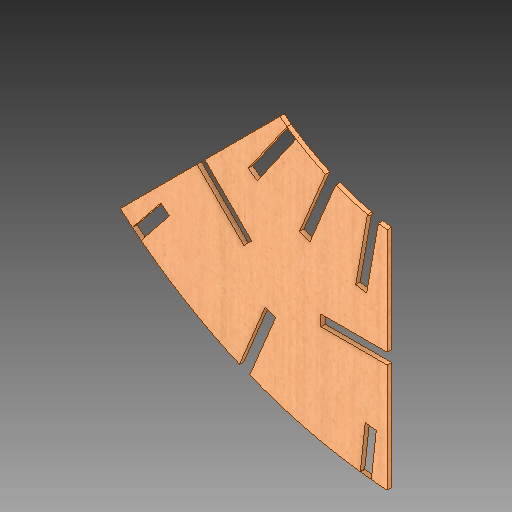
# Autodesk Inventor part: internalSupportTop5
Saved by Autodesk Inventor 2019 (Build 230136000, 136)
## iProperties
Company: FABLAB Torino
Created: 2019-01-11
Part Number: internalSupportTop5
Material: Wood (Cherry)
Document SubType Name: Modeling
Designer: Giancarlo
Density: 0.63 g/cm^3
Appearance: Cherry - Natural Low Gloss
Description: MultiLayer 10mm
Author: Giancarlo
Title: La Panca - Flower Vase
Subject: Construction MOld
Autodesk Inventor part; units mm, degrees
ref_plane "YZ Plane" through (0, 0, 0) normal (1, 0, 0) x (0, 1, 0)
ref_plane "XZ Plane" through (0, 0, 0) normal (0, 1, 0) x (-1, 0, 0)
ref_plane "Work Plane1" through (0, 0, 0) normal (0, 0, 1) x (1, 0, 0)
sketch "Sketch1" plane through (0, 0, 0) normal (0, 0, 1) x (1, 0, 0)
  line L0 (13.372447, 117.409014) -> (-9.931154, 61.149144)
  line L1 (13.372447, 117.409014) -> (4.133652, 121.235848)
  line L2 (-19.16995, 64.975978) -> (4.133652, 121.235848)
  line L3 (-9.931154, 61.149144) -> (-19.16995, 64.975978)
  line L4 (-22.457521, 135.166057) -> (-57.338279, 85.250516)
  line L5 (-22.457521, 135.166057) -> (-30.654475, 140.894052)
  line L6 (-65.535233, 90.978511) -> (-30.654475, 140.894052)
  line L7 (-57.338279, 85.250516) -> (-65.535233, 90.978511)
  line L8 (51.895734, 106.882533) -> (41.300176, 46.916168)
  line L9 (51.895734, 106.882533) -> (42.048271, 108.622498)
  line L10 (31.452714, 48.656133) -> (42.048271, 108.622498)
  line L11 (41.300176, 46.916168) -> (31.452714, 48.656133)
  line L12 (59.884796, 0) -> (0, 0)
  line L13 (59.884796, 0) -> (59.884796, 10)
  line L14 (0, 10) -> (59.884796, 10)
  line L15 (0, 0) -> (0, 10)
  line L16 (32.552055, -95.175797) -> (40.182275, -56.162387)
  line L17 (32.552055, -95.175797) -> (42.366116, -97.095226)
  line L18 (49.996336, -58.081815) -> (42.366116, -97.095226)
  line L19 (40.182275, -56.162387) -> (49.996336, -58.081815)
  line L20 (-81.40859, -85.281526) -> (-58.104996, -29.021673) construction
  line L21 (-81.40859, -85.281526) -> (-72.169794, -89.10836) construction
  line L22 (-48.8662, -32.848507) -> (-72.169794, -89.10836) construction
  line L23 (-58.104996, -29.021673) -> (-48.8662, -32.848507) construction
  line L24 (-167.86588, -9.726604) -> (-145.674595, 23.255452)
  line L25 (-167.86588, -9.726604) -> (-159.56905, -15.308952)
  line L26 (-137.377765, 17.673104) -> (-159.56905, -15.308952)
  line L27 (-145.674595, 23.255452) -> (-137.377765, 17.673104)
  line L28 (-104.69372, 78.180407) -> (-62.348775, 35.835462)
  line L29 (-104.69372, 78.180407) -> (-111.764788, 71.10934)
  line L30 (-69.419842, 28.764394) -> (-111.764788, 71.10934)
  line L31 (-62.348775, 35.835462) -> (-69.419842, 28.764394)
  line L32 (-180.237743, 2.642849) -> (-37.752284, 145.128308)
  spline S0 degree 3 poles (-37.139568, 145.91753) (-18.552876, 131.489971) (2.614229, 120.396776) (25.054803, 113.322882) (36.445472, 109.732226) (48.160059, 107.16983) (60.009605, 105.677025) knots -0.97612264 -0.97612264 -0.97612264 -0.97612264 -0.3444896 -0.3444896 -0.3444896 -0.02387736 -0.02387736 -0.02387736 -0.02387736
  line L33 (59.884796, 104.685705) -> (59.884796, -96.819163)
  spline S1 degree 3 poles (59.82253, -97.816466) (20.096664, -95.333409) (-19.252312, -86.903301) (-56.508733, -72.893707) (-93.770493, -58.882105) (-128.929435, -39.293038) (-160.452152, -14.980855) (-167.4509, -9.583006) (-174.271437, -3.954097) (-180.898913, 1.893621) knots -0.98831732 -0.98831732 -0.98831732 -0.98831732 -0.54882683 -0.54882683 -0.54882683 -0.10927338 -0.10927338 -0.10927338 -0.01168268 -0.01168268 -0.01168268 -0.01168268
  line L34 (-180.799713, 1.939457) -> (-37.031765, 145.707406)
  line L35 (59.784796, 105.604672) -> (59.784796, -97.71391)
  line L36 (-73.44623, -66.058689) -> (-50.142636, -9.798837)
  line L37 (-73.44623, -66.058689) -> (-64.207435, -69.885524)
  line L38 (-40.903841, -13.625671) -> (-64.207435, -69.885524)
  line L39 (-50.142636, -9.798837) -> (-40.903841, -13.625671)
  spline S2 degree 5 poles (-37.031765, 145.707405) (-28.648117, 139.214284) (-19.827811, 133.285293) (-10.628004, 127.950048) (8.422736, 118.525047) (28.553837, 111.703779) (38.836091, 108.983045) (49.264919, 106.940709) (59.784794, 105.604656) knots 0 0 0 0 0 0 0.49999712 0.49999712 0.49999712 1 1 1 1 1 1
  spline S3 degree 5 poles (59.784796, -97.713911) (42.142365, -96.609564) (24.561956, -94.525888) (7.112781, -91.482645) (-27.389088, -83.49215) (-60.810678, -71.774207) (-77.179784, -64.98315) (-109.100197, -49.642466) (-139.151316, -30.902327) (-153.646816, -20.722937) (-167.542932, -9.753367) (-180.799711, 1.939459) knots 0 0 0 0 0 0 0.33327801 0.33327801 0.33327801 0.66672126 0.66672126 0.66672126 1 1 1 1 1 1
  dimension "d0" = 0.1
  dimension "d8" = 0.1
  dimension "d1" = 0.1
  dimension "d2" = 0.1
  constraints: 4 end point, 2 parallel, 6 other
  measures "d1" distance between parallel lines of L32 L34
  measures "d2" distance between parallel lines of L33 L35
sketch "Sketch1 outline for Extrusion1" plane through (0, 0, 0) normal (0, 0, 1) x (1, 0, 0)
  spline S0 degree 5 poles (-37.031765, 145.707405) (-28.648117, 139.214284) (-19.827811, 133.285293) (-10.628004, 127.950048) (8.422736, 118.525047) (28.553837, 111.703779) (38.836091, 108.983045) (49.264919, 106.940709) (59.784794, 105.604656) knots 0 0 0 0 0 0 0.49999712 0.49999712 0.49999712 1 1 1 1 1 1
  line L0 (59.784794, 105.604656) -> (59.784796, -97.71391)
  spline S1 degree 5 poles (59.784796, -97.71391) (42.142365, -96.609564) (24.561956, -94.525888) (7.112781, -91.482645) (-27.389088, -83.49215) (-60.810678, -71.774207) (-77.179784, -64.98315) (-109.100197, -49.642466) (-139.151316, -30.902327) (-153.646816, -20.722937) (-167.542932, -9.753367) (-180.799711, 1.939459) knots 0 0 0 0 0 0 0.33327801 0.33327801 0.33327801 0.66672126 0.66672126 0.66672126 1 1 1 1 1 1
  line L1 (-180.799711, 1.939459) -> (-37.031765, 145.707405)
extrude "Extrusion1" add sketch "Sketch1 outline for Extrusion1" against normal blind 4
sketch "Sketch3" plane through (0, 0, 0) normal (0, 0, 1) x (1, 0, 0)
  line L0 (51.895734, 106.882533) -> (41.300176, 46.916168)
  line L1 (51.895734, 106.882533) -> (42.048271, 108.622498)
  line L2 (31.452714, 48.656133) -> (42.048271, 108.622498)
  line L3 (41.300176, 46.916168) -> (31.452714, 48.656133)
  line L4 (-9.931154, 61.149144) -> (-19.16995, 64.975978)
  line L5 (13.372447, 117.409014) -> (-9.931154, 61.149144)
  line L6 (-19.16995, 64.975978) -> (4.133652, 121.235848)
  line L7 (13.372447, 117.409014) -> (4.133652, 121.235848)
  line L8 (-22.457521, 135.166057) -> (-57.338279, 85.250516)
  line L9 (-22.457521, 135.166057) -> (-30.654475, 140.894052)
  line L10 (-65.535233, 90.978511) -> (-30.654475, 140.894052)
  line L11 (-57.338279, 85.250516) -> (-65.535233, 90.978511)
  line L12 (-73.44623, -66.058689) -> (-50.142636, -9.798837)
  line L13 (-73.44623, -66.058689) -> (-64.207435, -69.885524)
  line L14 (-40.903841, -13.625671) -> (-64.207435, -69.885524)
  line L15 (-50.142636, -9.798837) -> (-40.903841, -13.625671)
  line L16 (59.884796, 0) -> (0, 0)
  line L17 (0, 0) -> (0, 10)
  line L18 (0, 10) -> (59.884796, 10)
  line L19 (59.884796, 0) -> (59.884796, 10)
  line L20 (-69.419842, 28.764394) -> (-111.764788, 71.10934)
  line L21 (-104.69372, 78.180407) -> (-62.348775, 35.835462)
  line L22 (-62.348775, 35.835462) -> (-69.419842, 28.764394)
  line L23 (-104.69372, 78.180407) -> (-111.764788, 71.10934)
  line L24 (35.560087, -95.458706) -> (40.061177, -54.953661)
  line L25 (35.560087, -95.458706) -> (45.49891, -96.56315)
  line L26 (50, -56.058105) -> (45.49891, -96.56315)
  line L27 (40.061177, -54.953661) -> (50, -56.058105)
  line L28 (-169.884357, -7.34848) -> (-144.425716, 24.475663)
  line L29 (-169.884357, -7.34848) -> (-162.075588, -13.595329)
  line L30 (-136.616947, 18.228814) -> (-162.075588, -13.595329)
  line L31 (-144.425716, 24.475663) -> (-136.616947, 18.228814)
extrude "Extrusion3" cut sketch "Sketch3" against normal through all
body "Solid1"
